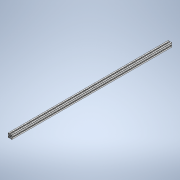
# Autodesk Inventor part: Perfil-de-aluminio-0001-001
Saved by Autodesk Inventor 2020.1 (Build 241239000, 239)
## iProperties
Created: 2024-04-05
Part Number: Perfil-de-aluminio-0001-001
Material: Generic
Document SubType Name: Modeling
Designer: MiguelBarbosa
Density: 1 g/cm^3
Appearance: Default
Author: MiguelBarbosa
Autodesk Inventor part; units mm, degrees
sketch "Sketch1" plane through (0, 0, 0) normal (0, 0, 1) x (1, 0, 0)
  circle A0 centre (0, 0) radius 6 construction
  circle A1 centre (0, 0) radius 7 construction
  line L0 (-1.3656, 6.8655) -> (0, 0) construction
  line L1 (0, 7) -> (0, 0) construction
  line L2 (-1.3656, 6.8655) -> (-1.1705, 5.8847)
  line L3 (1.1705, 5.8847) -> (1.3656, 6.8655)
  arc A2 (1.1705, 5.8847) -> (-1.1705, 5.8847) centre (0, 0) ccw
  arc A3 (-1.3656, 6.8655) -> (-3.889, 5.8203) centre (0, 0) ccw
  line L4 (-3.889, 5.8203) -> (0, 0) construction
  line L5 (-3.3334, 4.9888) -> (-3.889, 5.8203)
  arc A4 (-3.3334, 4.9888) -> (-4.9888, 3.3334) centre (0, 0) ccw
  line L6 (-5.8203, 3.889) -> (-4.9888, 3.3334)
  arc A5 (-5.8203, 3.889) -> (-6.8655, 1.3656) centre (0, 0) ccw
  line L7 (-5.8847, 1.1705) -> (-6.8655, 1.3656)
  arc A6 (-5.8847, 1.1705) -> (-5.8847, -1.1705) centre (0, 0) ccw
  line L8 (-6.8655, -1.3656) -> (-5.8847, -1.1705)
  arc A7 (-6.8655, -1.3656) -> (-5.8203, -3.889) centre (0, 0) ccw
  line L9 (-4.9888, -3.3334) -> (-5.8203, -3.889)
  arc A8 (-4.9888, -3.3334) -> (-3.3334, -4.9888) centre (0, 0) ccw
  line L10 (-3.889, -5.8203) -> (-3.3334, -4.9888)
  arc A9 (-3.889, -5.8203) -> (-1.3656, -6.8655) centre (0, 0) ccw
  line L11 (-1.1705, -5.8847) -> (-1.3656, -6.8655)
  arc A10 (-1.1705, -5.8847) -> (1.1705, -5.8847) centre (0, 0) ccw
  line L12 (1.3656, -6.8655) -> (1.1705, -5.8847)
  arc A11 (1.3656, -6.8655) -> (3.889, -5.8203) centre (0, 0) ccw
  line L13 (3.3334, -4.9888) -> (3.889, -5.8203)
  arc A12 (3.3334, -4.9888) -> (4.9888, -3.3334) centre (0, 0) ccw
  line L14 (5.8203, -3.889) -> (4.9888, -3.3334)
  arc A13 (5.8203, -3.889) -> (6.8655, -1.3656) centre (0, 0) ccw
  line L15 (5.8847, -1.1705) -> (6.8655, -1.3656)
  arc A14 (5.8847, -1.1705) -> (5.8847, 1.1705) centre (0, 0) ccw
  line L16 (6.8655, 1.3656) -> (5.8847, 1.1705)
  arc A15 (6.8655, 1.3656) -> (5.8203, 3.889) centre (0, 0) ccw
  line L17 (4.9888, 3.3334) -> (5.8203, 3.889)
  arc A16 (4.9888, 3.3334) -> (3.3334, 4.9888) centre (0, 0) ccw
  line L18 (3.889, 5.8203) -> (3.3334, 4.9888)
  arc A17 (3.889, 5.8203) -> (1.3656, 6.8655) centre (0, 0) ccw
  line L19 (-20.9, 14.1) -> (-14.1, 14.1) construction
  line L20 (-14.1, 14.1) -> (-14.1, 20.9) construction
  line L21 (-14.1, 20.9) -> (-20.9, 20.9) construction
  line L22 (-20.9, 20.9) -> (-20.9, 14.1) construction
  line L23 (-20.9, 14.1) -> (-14.1, 20.9) construction
  line L24 (-14.1, 14.1) -> (-20.9, 20.9) construction
  line L25 (-13.5, 21.5) -> (-21.5, 21.5) construction
  line L26 (-21.5, 21.5) -> (-21.5, 13.5) construction
  line L27 (-21.5, 13.5) -> (-13.5, 13.5) construction
  line L28 (-13.5, 13.5) -> (-13.5, 21.5) construction
  line L29 (-13.5, 21.5) -> (-21.5, 13.5) construction
  line L30 (-21.5, 21.5) -> (-13.5, 13.5) construction
  line L31 (-16, 21.5) -> (-16, 20.9)
  line L32 (-16, 20.9) -> (-19, 20.9)
  line L33 (-16, 21.5) -> (-13.5, 21.5)
  line L34 (-13.5, 21.5) -> (-13.5, 19)
  line L35 (-13.5, 19) -> (-14.1, 19)
  line L36 (-14.1, 19) -> (-14.1, 16)
  line L37 (-14.1, 16) -> (-13.5, 16)
  line L38 (-13.5, 16) -> (-13.5, 13.5) construction
  line L39 (-13.5, 13.5) -> (-16, 13.5) construction
  line L40 (-16, 13.5) -> (-16, 14.1)
  line L41 (-16, 14.1) -> (-19, 14.1)
  line L42 (-19, 14.1) -> (-19, 13.5)
  line L43 (-19, 13.5) -> (-21.5, 13.5)
  line L44 (-21.5, 13.5) -> (-21.5, 16)
  line L45 (-21.5, 16) -> (-20.9, 16)
  line L46 (-20.9, 16) -> (-20.9, 19)
  line L47 (-20.9, 19) -> (-21.5, 19)
  line L48 (-21.5, 19) -> (-21.5, 21.5) construction
  line L49 (-19, 20.9) -> (-19, 21.5)
  line L50 (-19, 21.5) -> (-21.5, 21.5) construction
  line L51 (-17.5, 17.5) -> (17.5, 17.5) construction
  line L52 (-17.5, 17.5) -> (-17.5, -17.5) construction
  line L53 (-25, 25) -> (25, 25) construction
  line L54 (-25, 25) -> (-25, -25) construction
  line L55 (-25, 25) -> (-5.1, 25) construction
  line L56 (5.1, 25) -> (-5.1, 25) construction
  line L57 (-5.1, 25) -> (-7.1, 25) construction
  line L58 (-7.1, 25) -> (-7.1, 23)
  line L59 (-7.1, 23) -> (-5.1, 23)
  line L60 (-5.1, 23) -> (-5.1, 25) construction
  line L61 (-5.1, 25) -> (-7.1, 23) construction
  line L62 (-7.1, 25) -> (-5.1, 23) construction
  line L63 (-7.1, 25) -> (-25, 25) construction
  line L64 (-25, 25) -> (-25, 5.1) construction
  line L65 (-25, 5.1) -> (-23, 5.1) construction
  line L66 (-23, 5.1) -> (-23, 7.1)
  line L67 (-23, 7.1) -> (-25, 7.1)
  line L68 (-25, 7.1) -> (-25, 5.1) construction
  line L69 (-25, 5.1) -> (-23, 7.1) construction
  line L70 (-23, 5.1) -> (-25, 7.1) construction
  line L71 (-25, 25) -> (-25, 7.1) construction
  line L72 (-5.1, 23) -> (-5.1, 19)
  line L73 (-5.1, 19) -> (-10, 19)
  line L74 (-10, 19) -> (-10, 12) construction
  line L75 (-10, 12) -> (0, 12) construction
  circle A18 centre (0, 0) radius 12
  line L76 (-23, 5.1) -> (-19, 5.1)
  line L77 (-19, 5.1) -> (-19, 10)
  line L78 (-19, 10) -> (-12, 10) construction
  line L79 (-12, 10) -> (-12, 0) construction
  line L80 (-13.5, 21.5) -> (-13.5, 25) construction
  line L81 (-10, 19) -> (-13.5, 19) construction
  arc A19 (-10, 15.5) -> (-4.0387, 11.3) centre (-5.5398, 15.5) ccw
  line L82 (-10, 19) -> (-10, 15.5)
  arc A20 (-11.3, 4.0387) -> (-15.5, 10) centre (-15.5, 5.5398) ccw
  line L83 (-15.5, 10) -> (-19, 10)
  arc A21 (-23, 25) -> (-25, 23) centre (-23, 23) ccw
  line L84 (-23, 25) -> (-7.1, 25)
  line L85 (-25, 23) -> (-25, 7.1)
  arc A22 (-14.5, 13.5) -> (-13.5, 14.5) centre (-14.5, 14.5) ccw
  line L86 (-13.5, 16) -> (-13.5, 14.5)
  line L87 (-16, 13.5) -> (-14.5, 13.5)
  arc A23 (-20.5, 21.5) -> (-21.5, 20.5) centre (-20.5, 20.5) ccw
  line L88 (-20.5, 21.5) -> (-19, 21.5)
  line L89 (-21.5, 20.5) -> (-21.5, 19)
  point P0 (-17.5, 17.5)
  point P1 (-17.5, 17.5)
  point P2 (-17.5, 21.5)
  point P3 (-17.5, 20.9)
  point P4 (0, 17.5)
  point P5 (-17.5, 0)
  point P6 (0, 25)
  point P7 (-25, 0)
  point P8 (-6.1, 24)
  point P9 (-24, 6.1)
  point P10 (3.889, -5.8203)
  point P11 (-6.8655, 1.3656)
  dimension "d12" = 12
  dimension "d13" = 14
  dimension "d18" = 360
  dimension "d20" = 22.5
  dimension "d23" = 6.8
  dimension "d24" = 8
  dimension "d26" = 3
  dimension "d27" = 35
  dimension "d28" = 50
  dimension "d30" = 10.2
  dimension "d32" = 6
  dimension "d33" = 13
  dimension "d35" = 2
  dimension "d39" = 1
  dimension "d40" = 2
  constraints: 180 end point, 51 point on circle, 35 perpendicular, 25 point on line, 24 centre point, 22 midpoint, 13 horizontal, 13 vertical, 12 tangent, 8 coincident, 8 parallel, 5 collinear, 4 vertical alignment, 2 horizontal alignment, 1 equal radius, 90 other
  measures "d12" diameter of A0
  measures "d13" diameter of A1
  measures "d20" angle of L0 L4
  measures "d23" distance of L20.end L21.end
  measures "d24" distance of L25.start L25.end
  measures "d26" distance of L31.end L32.end
  measures "d27" distance of L51.start L51.end
  measures "d28" distance of L53.start L53.end
  measures "d30" distance of L56.start L56.end
  measures "d32" distance from line of L53 L72.end
  measures "d33" distance from line of L75.end L55
  measures "d35" distance of L58.end L59.end
  measures "d39" radius of A23
  measures "d40" radius of A21
extrude "Extrusion1" add sketch "Sketch1" along normal mid plane 2000 contours A18
extrude "Extrusion2" add sketch "Sketch1" along normal mid plane 2000 contours L58 L59 L72 L73 L82 A19 A18 A20 L83 L77 L76 L66 L67 L85 A21 L84
pattern_circular "Circular Pattern1" count 4 over 360 about axis through (0, 0, 0) along (0, 0, 1) of "Extrusion2"
body "Solid1"
